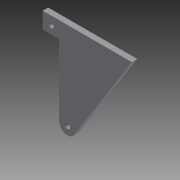
# Autodesk Inventor part: Elevator Latch
Saved by Autodesk Inventor 2015 (Build 190159000, 159)
## iProperties
Created: 2015-01-25
Part Number: Elevator Latch
Material: Generic
Document SubType Name: Modeling
Designer: chapale16
Density: 1 g/cm^3
Appearance: Default
Author: chapale16
Autodesk Inventor part; units mm, degrees
ref_plane "YZ Plane" through (0, 0, 0) normal (1, 0, 0) x (0, 1, 0)
ref_plane "XZ Plane" through (0, 0, 0) normal (0, 1, 0) x (-1, 0, 0)
ref_plane "XY Plane" through (0, 0, 0) normal (0, 0, 1) x (1, 0, 0)
sketch "Sketch1" plane through (0, 0, 0) normal (0, 0, 1) x (1, 0, 0)
  line L0 (0, 0) -> (103.505, 0)
  line L1 (103.505, 0) -> (103.505, -19.05)
  line L2 (103.505, -19.05) -> (0, -19.05)
  line L3 (0, -19.05) -> (0, 0)
  line L4 (19.05, 0) -> (19.05, -101.6)
  circle A0 centre (28.575, -101.6) radius 9.525
  line L5 (103.505, 0) -> (36.6455, -106.659)
  circle A1 centre (28.575, -101.6) radius 3.175
  circle A2 centre (9.525, -9.525) radius 3.175
  dimension "d0" = 103.505
  dimension "d1" = 19.05
  dimension "d2" = 101.6
  dimension "d3" = 6.35
  dimension "d4" = 6.35
  constraints: 12 end point, 3 centre point, 2 parallel, 2 point on circle, 1 coincident, 1 horizontal, 1 perpendicular, 1 point on line, 1 tangent, 1 vertical
  measures "d0" distance of L1.end L2.end
  measures "d1" distance of L0.end L1.end
  measures "d2" distance of L4.start L4.end
  measures "d3" diameter of A1
  measures "d4" diameter of A2
extrude "Extrusion1" add sketch "Sketch1" along normal blind 3.175
sketch "Sketch2" plane through (0, 0, 3.175) normal (0, 0, 1) x (1, 0, 0)
  line L0 (91.5634, -19.05) -> (103.505, 0)
  line L1 (103.505, 0) -> (141.6118, -29.0679)
  line L2 (141.6118, -29.0679) -> (106.1951, -49.8481)
  line L3 (106.1951, -49.8481) -> (91.5634, -19.05)
  point P0 (0, 0)
  constraints: 8 end point
extrude "Extrusion2" cut sketch "Sketch2" against normal blind 6.35
sketch "Sketch3" plane through (0, 0, 3.175) normal (0, 0, 1) x (1, 0, 0)
  line L0 (19.05, -19.05) -> (22.3566, -51.6435)
  line L1 (22.3566, -51.6435) -> (19.05, -54.458)
  line L2 (19.05, -54.458) -> (19.05, -19.05)
  line L3 (0, -19.05) -> (19.05, -19.05) projected
  point P0 (0, 0)
  constraints: 6 end point, 1 perpendicular
extrude "Extrusion3" cut sketch "Sketch3" against normal blind 3.175
body "Solid1"
